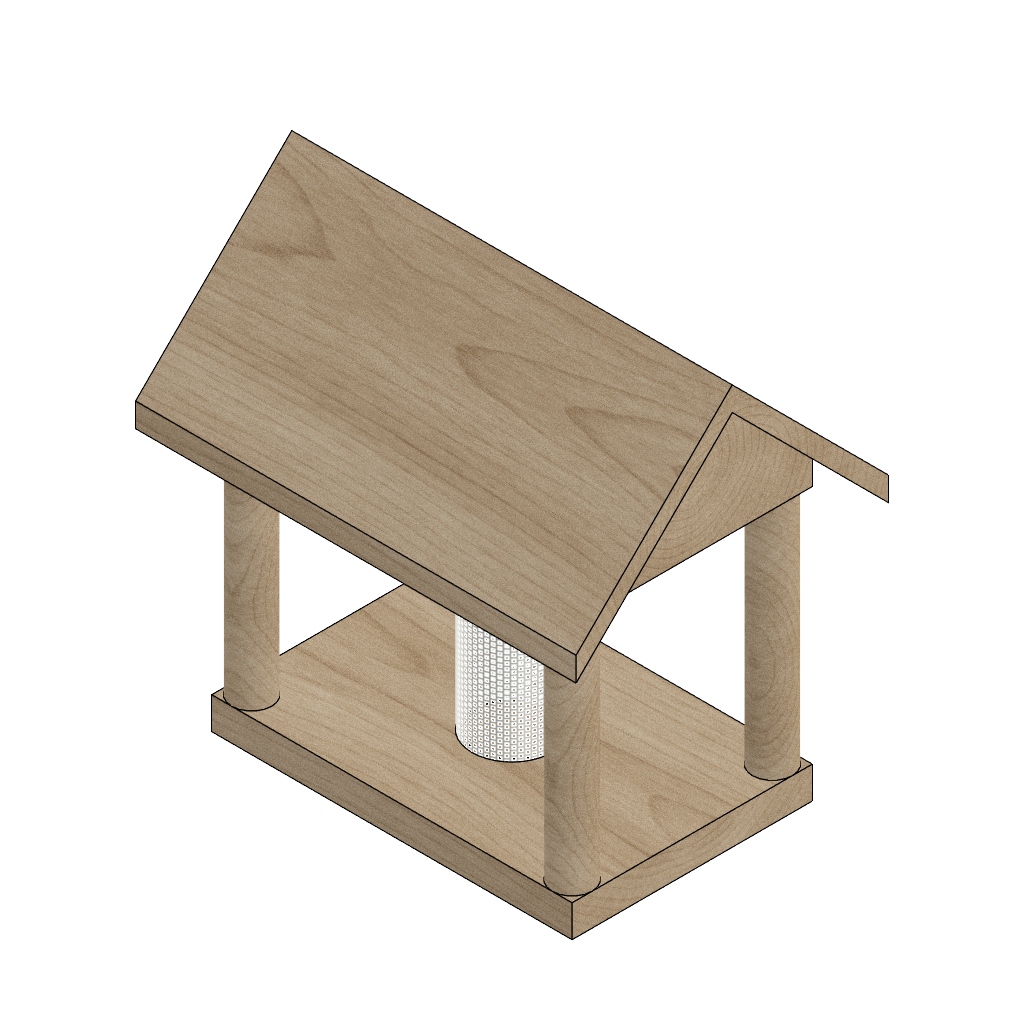
Vogelhaus (Autodesk Fusion 360 design; units mm, degrees)
part number: 2026-02-16-19-10-45-756
Autodesk Fusion 360 part; units mm, degrees
sketch "Sketch1" plane through (0, 0, 0) normal (0, 0, 1) x (1, 0, 0)
  line L0 (0, 0) -> (450, 0)
  line L1 (450, 0) -> (450, 300)
  line L2 (450, 300) -> (0, 300)
  line L3 (0, 300) -> (0, 0)
  line L4 (0, 300) -> (50, 300)
  line L5 (50, 300) -> (50, 250)
  line L6 (50, 250) -> (0, 250)
  line L7 (0, 250) -> (0, 300)
  line L8 (225, 300) -> (225, 0) construction
  line L9 (450, 150) -> (0, 150) construction
  line L10 (50, 0) -> (50, 50)
  line L11 (50, 50) -> (0, 50)
  line L12 (400, 0) -> (400, 50)
  line L13 (400, 50) -> (450, 50)
  line L14 (400, 250) -> (450, 250)
  line L15 (400, 300) -> (400, 250)
  circle A0 centre (225, 150) radius 50
  circle A1 centre (225, 150) radius 45
  circle A2 centre (25, 25) radius 25
  circle A3 centre (25, 275) radius 25
  circle A4 centre (425, 275) radius 25
  circle A5 centre (425, 25) radius 25
  dimension "d1" = 450
  dimension "d2" = 300
  dimension "d5" = 50
  dimension "d6" = 50
  dimension "d9" = 100
  dimension "d12" = 90
  constraint horizontal L0
  constraint vertical L1
  constraint horizontal L2
  constraint vertical L3
  constraint coincident L0.start L3.end
  constraint horizontal L4
  constraint vertical L5
  constraint horizontal L6
  constraint vertical L7
  constraint midpoint L2 L8.start
  constraint midpoint L0 L8.end
  constraint midpoint L1 L9.start
  constraint midpoint L3 L9.end
  constraint symmetric L4.end L9 L10.start
  constraint symmetric L5.end L9 L10.end
  constraint symmetric L6.end L9 L11.end
  constraint symmetric L4.end L8 L15.start
  constraint symmetric L5.end L8 L14.start
  constraint symmetric L6.end L8 L14.end
  constraint symmetric L8 L10.start L12.start
  constraint symmetric L8 L10.end L12.end
  constraint symmetric L8 L11.end L13.end
  constraint midpoint L9 A0.centre
  constraint concentric A0 A1
  constraint tangent L11 A2
  constraint tangent L3 A2
  constraint tangent L0 A2
  constraint symmetric L9 A2 A3
  constraint symmetric L8 A2 A5
  constraint symmetric L8 A3 A4
  measures "d1" distance of L0.start L0.end
  measures "d2" distance of L0.start L2.end
  measures "d5" distance of L2.end L4.end
  measures "d6" distance of L2.end L6.end
  measures "d9" diameter of A0
  measures "d12" diameter of A1
extrude "Extrude1" add sketch "Sketch1" against normal blind 40 contours L0 L1 L2 L3 L5 L6 L10 L11 L12 L13 L14 L15 | L0 L10 A2 | L0 L12 A5 | L0 L3 A2 | A2 | L10 L11 A2 | L0 L1 A5 | A5 | L12 L13 A5 | L3 L11 A2 | L1 L13 A5 | L3 L6 L7 A3 | L1 L14 A4 | L2 L3 L4 L7 A3 | A3 | L5 L6 A3 | L1 L2 A4 | A4 | L14 L15 A4 | L2 L4 L5 A3 | L2 L15 A4 | A0 | A1 makes body 1
extrude "Extrude2" add sketch "Sketch1" along normal blind 300 contours A2 | A5 | A3 | A4 bodies 1
sketch "Sketch2" plane through (0, 0, 300) normal (0, 0, 1) x (-1, 0, 0)
  circle A0 centre (-25, -275) radius 25
  circle A1 centre (-25, -25) radius 25
  circle A2 centre (-425, -275) radius 25
  circle A3 centre (-425, -25) radius 25
extrude "Extrude4" add sketch "Sketch1" along normal blind 300 separate body contours A0 makes body 2
sketch "Sketch3" plane through (0, 0, 0) normal (0, -1, 0) x (1, 0, 0)
  line L0 (0, 0) -> (50, 0)
  line L1 (50, 0) -> (50, 300)
  line L2 (50, 300) -> (0, 300)
  line L3 (0, 300) -> (0, 0)
  circle A0 centre (225, 45) radius 20
  circle A1 centre (225, 115) radius 20
  circle A2 centre (225, 185) radius 20
  circle A3 centre (225, 255) radius 20
  line L4 (225, 0) -> (225, 45) construction
  line L5 (450, 0) -> (0, 0)
  line L6 (0, 0) -> (0, -40)
  line L7 (0, -40) -> (450, -40)
  line L8 (450, -40) -> (450, 0)
  point P0 (225, 0)
  dimension "d15" = 40
  dimension "d20" = 0
  dimension "d21" = 140
  dimension "d24" = 45
  dimension "d55" = 0
  dimension "d56" = 70
  constraint coincident P0 L4.start
  constraint coincident A0.centre L4.end
  constraint vertical L4
  measures "d15" diameter of A0
  measures "d24" distance of A0.centre P0
extrude "Extrude12" [suppressed]
sketch "Sketch4" plane through (450, 0, 0) normal (1, 0, 0) x (0, 1, 0)
  line L0 (0, 0) -> (300, 0)
  line L1 (300, 300) -> (0, 300)
  line L2 (0, 300) -> (0, 0)
  circle A0 centre (150, 40) radius 20
  circle A1 centre (150, 110) radius 20
  circle A2 centre (150, 180) radius 20
  circle A3 centre (150, 250) radius 20
  line L3 (300, 0) -> (300, 300)
  line L4 (25, 0) -> (0, 0)
  line L5 (0, 0) -> (0, -40)
  line L6 (0, -40) -> (300, -40)
  line L7 (300, -40) -> (300, 0)
  line L8 (300, 0) -> (275, 0)
  line L9 (275, 0) -> (25, 0)
  point P0 (150, 0)
  dimension "d25" = 40
  dimension "d26" = 40
  dimension "d29" = 0
  dimension "d30" = 140
  dimension "d61" = 0
  dimension "d62" = 70
  measures "d25" diameter of A0
  measures "d26" distance of A0.centre P0
extrude "Extrude13" [suppressed]
sketch "Sketch5" plane through (0, 0, 300) normal (0, 0, 1) x (-1, 0, 0)
  line L0 (0, 0) -> (-450, 0)
  line L1 (-450, 0) -> (-450, -300)
  line L2 (-450, -300) -> (0, -300)
  line L3 (0, -300) -> (0, 0)
  line L4 (-400, 0) -> (-425, 0)
  line L5 (-50, -300) -> (-25, -300)
  arc A0 (-25, -300) -> (-50, -275) centre (-25, -275) ccw
  line L6 (-50, -275) -> (-50, -300)
  circle A1 centre (-425, -275) radius 25
  circle A2 centre (-25, -25) radius 25
  arc A3 (-425, 0) -> (-400, -25) centre (-425, -25) ccw
  line L7 (-400, -25) -> (-400, 0)
  circle A4 centre (-225, -150) radius 50
  circle A5 centre (-425, -275) radius 25
  point P0 (-450, -300)
  constraint horizontal L0
  constraint vertical L1
  constraint horizontal L2
  constraint vertical L3
  constraint coincident P0 L1.end
extrude "Extrude8" add sketch "Sketch5" along normal blind 30 separate body contours L0 L4 A3 L7 | L0 L1 L2 L3 A0 L6 A1 A2 A3 L7 A5 | L0 L1 A3 | L0 L3 A2 | A2 | L1 L2 A1 A5 | A1 A5 | L2 L3 A0 | L2 L5 A0 L6 | A4 makes body 3
sketch "Sketch7" plane through (450, 0, 0) normal (1, 0, 0) x (0, 1, 0)
  line L0 (300, 300) -> (300, 330)
  line L1 (300, 330) -> (0, 330)
  line L2 (0, 330) -> (0, 300)
  line L3 (0, 330) -> (207.3852, 330) construction
  line L4 (345, 285) -> (149.1978, 480.8022)
  line L5 (300, 330) -> (87.2017, 330) construction
  line L6 (150, 300) -> (150, 530) construction
  line L7 (-45, 285) -> (150.8022, 480.8022)
  line L8 (-45, 285) -> (-45, 315.0528)
  line L9 (-45, 315.0528) -> (150, 510.0528)
  line L10 (345, 285) -> (345, 315.0528)
  line L11 (345, 315.0528) -> (150, 510.0528)
  line L12 (0, 300) -> (300, 300)
  dimension "d39" = 45
  constraint horizontal L3
  constraint coincident L1.end L2.start
  constraint horizontal L5
  constraint symmetric L4.end L6 L7.end
  constraint symmetric L4.start L6 L7.start
  constraint vertical L8
  constraint coincident L6 L9.end
  constraint parallel L7 L9
  constraint symmetric L6 L7.start L4.start
  constraint symmetric L6 L8.end L10.end
  constraint symmetric L6 L9.end L11.end
  measures "d39" angle of L4 L5
extrude "Extrude11" add sketch "Sketch7" along normal blind 50 and the other way blind 500 separate body contours L4 L7 L8 L9 L10 L11 makes body 4
sketch "Sketch8" plane through (0, 0, 330) normal (0, 0, 1) x (-1, 0, 0)
  line L0 (0, -300) -> (0, 0)
  line L1 (0, 0) -> (-450, 0)
  line L2 (-450, 0) -> (-450, -300)
  line L3 (-450, -300) -> (0, -300)
  line L4 (-450, -163.7778) -> (-420, -163.7778)
  line L5 (-420, -163.7778) -> (-420, -133.7778)
  line L6 (-420, -133.7778) -> (-450, -133.7778)
  line L7 (-450, -133.7778) -> (-450, -163.7778)
  line L8 (-450, -163.7778) -> (-450, -133.7778)
  dimension "d49" = 30
  dimension "d50" = 30
  constraint horizontal L4
  constraint vertical L5
  constraint horizontal L6
  constraint vertical L7
  constraint coincident L2 L4.start
  measures "d49" distance of L4.start L4.end
  measures "d50" distance of L4.start L6.end
extrude "Extrude14" add sketch "Sketch7" along normal blind -25 and the other way blind 0 contours L1 L4 L7 bodies 1 3
extrude "Extrude15" add sketch "Sketch7" against normal blind 30 from surface at -420 contours L1 L4 L7 bodies 1 4 3
sketch "Sketch15" plane through (0, 0, 330) normal (0, 0, 1) x (-1, 0, 0)
  line L0 (-30, -300) -> (-30, 0)
  line L1 (-425, 0) -> (-425, -300)
  line L2 (-420, -165) -> (-390, -165)
  line L3 (-390, -165) -> (-390, -135)
  line L4 (-390, -135) -> (-420, -135)
  line L5 (-420, -135) -> (-420, -165)
  line L6 (-30, 0) -> (-425, 0)
  line L7 (-425, -300) -> (-30, -300)
  dimension "d79" = 30
  dimension "d80" = 30
  dimension "d82" = 5
  constraint horizontal L2
  constraint vertical L3
  constraint horizontal L4
  constraint vertical L5
  measures "d79" distance of L2.start L2.end
  measures "d80" distance of L2.start L4.end
  measures "d82" distance of L1 L5
sketch "Sketch16" plane through (0, 0, 300) normal (0, 0, -1) x (1, 0, 0)
  line L0 (0, -300) -> (450, -300)
  line L1 (450, -300) -> (450, 0)
  line L2 (450, 0) -> (0, 0)
  line L3 (0, 0) -> (0, -300)
  line L4 (390, -165) -> (360, -165)
  line L5 (360, -165) -> (360, -135)
  line L6 (360, -135) -> (390, -135)
  line L7 (390, -135) -> (390, -165)
  dimension "d85" = 30
  dimension "d86" = 30
  dimension "d87" = 135
  dimension "d88" = 60
  constraint horizontal L4
  constraint vertical L5
  constraint horizontal L6
  constraint vertical L7
  measures "d85" distance of L4.start L4.end
  measures "d86" distance of L4.start L6.end
  measures "d87" distance of L1.end L6
  measures "d88" distance of L1 L7
loft "Loft3" cut profiles "Sketch16", "Sketch15" section 1 contours L4 L5 L6 L7 section 2 contours L2 L3 L4 L5 bodies 4 1
